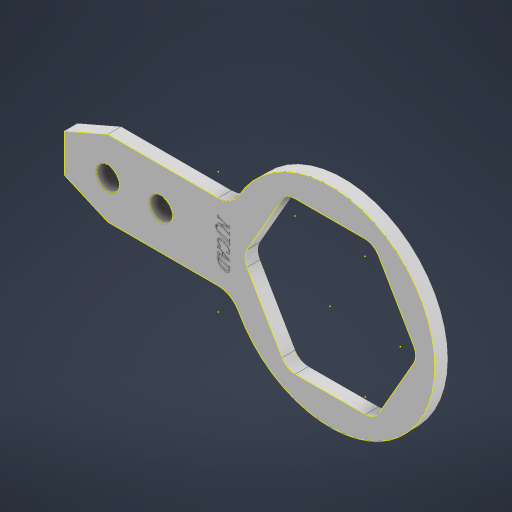
# Autodesk Inventor part: BICYCLE SPANNER
Saved by Autodesk Inventor 2023 (Build 270158000, 158)
## iProperties
Created: 2024-01-19
Part Number: BICYCLE SPANNER
Material: Generic
Document SubType Name: Modeling
Designer: User
Density: 1 g/cm^3
Appearance: Default
Author: User
Autodesk Inventor part; units mm, degrees
ref_plane "YZ Plane" through (0, 0, 0) normal (1, 0, 0) x (0, 1, 0)
ref_plane "XZ Plane" through (0, 0, 0) normal (0, 1, 0) x (-1, 0, 0)
ref_plane "XY Plane" through (0, 0, 0) normal (0, 0, 1) x (1, 0, 0)
sketch "Sketch1" plane through (0, 0, 0) normal (0, 0, 1) x (1, 0, 0)
  line L0 (25.3172, 36.0607) -> (43.8689, 4.105)
  line L1 (43.8881, -3.8949) -> (25.4895, -35.9391)
  line L2 (18.5709, -39.9557) -> (-18.3794, -40.0441)
  line L3 (-25.3172, -36.0607) -> (-43.8689, -4.105)
  line L4 (-43.8881, 3.8949) -> (-25.4895, 35.9391)
  line L5 (-18.5709, 39.9557) -> (18.3794, 40.0441)
  arc A0 (-48.3214, -26.2687) -> (-48.3214, 26.2687) centre (0, 0) ccw
  line L6 (-58.8643, 20) -> (-117, 20)
  line L7 (-58.8643, -20) -> (-117, -20)
  line L8 (-140, 10) -> (-140, -10)
  line L9 (-140, 0) -> (0, 0) construction
  line L10 (-117, 20) -> (-140, 10)
  line L11 (-140, -10) -> (-117, -20)
  arc A1 (-58.8643, 20) -> (-48.3214, 26.2687) centre (-58.8643, 32) ccw
  arc A2 (-48.3214, -26.2687) -> (-58.8643, -20) centre (-58.8643, -32) ccw
  arc A3 (-18.5709, 39.9557) -> (-25.4895, 35.9391) centre (-18.5518, 31.9557) ccw
  arc A4 (25.3172, 36.0607) -> (18.3794, 40.0441) centre (18.3985, 32.0441) ccw
  arc A5 (-43.8881, 3.8949) -> (-43.8689, -4.105) centre (-36.9503, -0.0885) ccw
  arc A6 (43.8881, -3.8949) -> (43.8689, 4.105) centre (36.9503, 0.0885) ccw
  arc A7 (18.5709, -39.9557) -> (25.4895, -35.9391) centre (18.5518, -31.9557) ccw
  arc A8 (-25.3172, -36.0607) -> (-18.3794, -40.0441) centre (-18.3985, -32.0441) ccw
  circle A9 centre (-117, 0) radius 6
  circle A10 centre (-89, 0) radius 6
  point P0 (22.9982, 40.0552)
  point P1 (46.1879, 0.1106)
  point P2 (23.1897, -39.9446)
  point P3 (-22.9982, -40.0552)
  point P4 (-46.1879, -0.1106)
  point P5 (-23.1897, 39.9446)
  point P6 (-0.0958, 39.9999)
  point P7 (0.0958, -39.9999)
  point P8 (-51.2348, -20)
  point P9 (-51.2348, 20)
  dimension "d1" = 79.9998
  dimension "d2" = 80
  dimension "d3" = 110
  dimension "d4" = 20
  dimension "d5" = 140
  dimension "d6" = 40
  dimension "d10" = 12
  dimension "d11" = 8
  dimension "d12" = 12
  dimension "d13" = 23
  dimension "d14" = 28
  constraints: 24 end point, 20 point on circle, 16 point on line, 16 tangent, 11 centre point, 7 equal radius, 3 horizontal, 3 midpoint, 2 coincident, 2 vertical alignment, 1 horizontal alignment, 1 vertical, 14 other
  measures "d1" vertical distance of point (-0.096, 40) point (0.096, -40)
  measures "d2" distance of point (46.188, 0.111) point (-22.998, -40.055)
  measures "d3" diameter of A0
  measures "d4" distance of L8.start L8.end
  measures "d5" distance of L9.start point (0, 0)
  measures "d6" distance between parallel lines of L7 L6
  measures "d10" radius of A1
  measures "d11" radius of A3
  measures "d12" diameter of A9
  measures "d13" horizontal distance of A9.centre L8.end
  measures "d14" distance of A10.centre A9.centre
extrude "Extrusion1" add sketch "Sketch1" along normal blind 7
sketch "Sketch2" plane through (0, 0, 7) normal (0, 0, 1) x (1, 0, 0)
  arc A0 (-48.3214, -26.2687) -> (-48.3214, 26.2687) centre (0, 0) ccw projected
  arc A1 (-58.8643, 20) -> (-48.3214, 26.2687) centre (-58.8643, 32) ccw projected
  line L0 (-58.8643, 20) -> (-117, 20) projected
  line L1 (-117, 20) -> (-140, 10) projected
  line L2 (-140, 10) -> (-140, -10) projected
  line L3 (-140, -10) -> (-117, -20) projected
  line L4 (-117, -20) -> (-58.8643, -20) projected
  arc A2 (-48.3214, -26.2687) -> (-58.8643, -20) centre (-58.8643, -32) ccw projected
  line L5 (-18.5709, 39.9557) -> (18.3794, 40.0441) projected
  arc A3 (25.3172, 36.0607) -> (18.3794, 40.0441) centre (18.3985, 32.0441) ccw projected
  line L6 (25.3172, 36.0607) -> (43.8689, 4.105) projected
  arc A4 (43.8881, -3.8949) -> (43.8689, 4.105) centre (36.9503, 0.0885) ccw projected
  line L7 (43.8881, -3.8949) -> (25.4895, -35.9391) projected
  arc A5 (18.5709, -39.9557) -> (25.4895, -35.9391) centre (18.5518, -31.9557) ccw projected
  line L8 (18.5709, -39.9557) -> (-18.3794, -40.0441) projected
  arc A6 (-25.3172, -36.0607) -> (-18.3794, -40.0441) centre (-18.3985, -32.0441) ccw projected
  line L9 (-25.3172, -36.0607) -> (-43.8689, -4.105) projected
  arc A7 (-43.8881, 3.8949) -> (-43.8689, -4.105) centre (-36.9503, -0.0885) ccw projected
  line L10 (-43.8881, 3.8949) -> (-25.4895, 35.9391) projected
  arc A8 (-18.5709, 39.9557) -> (-25.4895, 35.9391) centre (-18.5518, 31.9557) ccw projected
  circle A9 centre (-89, 0) radius 6 projected
  circle A10 centre (-117, 0) radius 6 projected
sketch "Sketch4" plane through (0, 0, 7) normal (0, 0, 1) x (1, 0, 0)
  line L0 (-52.8304, 12.3394) -> (-52.8304, -11.579) construction
  line L1 (-52.8304, -11.579) -> (-60.2146, -11.579) construction
  line L2 (-60.2146, -11.579) -> (-60.2146, 12.3394) construction
  line L3 (-60.2146, 12.3394) -> (-52.8304, 12.3394) construction
  line L4 (-57.6462, 8.2014) -> (-57.6462, 8.13)
  line L5 (-57.6462, 8.13) -> (-53.4725, 6.712)
  spline S0 degree 2 poles (-53.4725, 6.712) (-53.3298, 6.663) (-53.1871, 6.7611) (-53.1871, 6.9395) knots 0 0 0 1 2 2 2
  line L6 (-53.1871, 6.9395) -> (-53.1871, 7.2248)
  line L7 (-53.1871, 7.2248) -> (-52.9731, 7.149)
  line L8 (-52.9731, 7.149) -> (-52.9731, 5.7221)
  line L9 (-52.9731, 5.7221) -> (-53.1871, 5.7979)
  line L10 (-53.1871, 5.7979) -> (-53.1871, 6.0833)
  spline S1 degree 2 poles (-53.1871, 6.0833) (-53.1871, 6.226) (-53.3298, 6.449) (-53.4725, 6.498) knots 0 0 0 1 2 2 2
  line L11 (-53.4725, 6.498) -> (-59.0731, 8.402)
  line L12 (-59.0731, 8.402) -> (-59.0731, 8.6161)
  line L13 (-59.0731, 8.6161) -> (-53.7579, 9.5213)
  line L14 (-53.7579, 9.5213) -> (-53.7579, 9.5926)
  line L15 (-53.7579, 9.5926) -> (-58.5737, 11.2291)
  spline S2 degree 2 poles (-58.5737, 11.2291) (-58.7163, 11.2781) (-58.859, 11.1488) (-58.859, 11.0061) knots 0 0 0 1 2 2 2
  line L16 (-58.859, 11.0061) -> (-58.859, 10.7207)
  line L17 (-58.859, 10.7207) -> (-59.0731, 10.7921)
  line L18 (-59.0731, 10.7921) -> (-59.0731, 12.219)
  line L19 (-59.0731, 12.219) -> (-58.859, 12.1476)
  line L20 (-58.859, 12.1476) -> (-58.859, 11.8623)
  spline S3 degree 2 poles (-58.859, 11.8623) (-58.859, 11.6839) (-58.7163, 11.4922) (-58.5737, 11.4431) knots 0 0 0 1 2 2 2
  line L21 (-58.5737, 11.4431) -> (-53.4725, 9.7085)
  spline S4 degree 2 poles (-53.4725, 9.7085) (-53.3298, 9.6595) (-53.1871, 9.7576) (-53.1871, 9.9359) knots 0 0 0 1 2 2 2
  line L22 (-53.1871, 9.9359) -> (-53.1871, 10.15)
  line L23 (-53.1871, 10.15) -> (-52.9731, 10.0742)
  line L24 (-52.9731, 10.0742) -> (-52.9731, 9.0397)
  line L25 (-52.9731, 9.0397) -> (-57.6462, 8.2014)
  spline S5 degree 2 poles (-53.4725, 3.2161) (-53.3298, 3.1671) (-53.1871, 3.2652) (-53.1871, 3.4436) knots 0 0 0 1 2 2 2
  line L26 (-53.1871, 3.4436) -> (-53.1871, 4.2997)
  line L27 (-53.1871, 4.2997) -> (-52.9731, 4.2239)
  line L28 (-52.9731, 4.2239) -> (-52.9731, 1.2987)
  line L29 (-52.9731, 1.2987) -> (-53.1871, 1.3745)
  line L30 (-53.1871, 1.3745) -> (-53.1871, 2.2307)
  spline S6 degree 2 poles (-53.1871, 2.2307) (-53.1871, 2.3734) (-53.3298, 2.5963) (-53.4725, 2.6454) knots 0 0 0 1 2 2 2
  line L31 (-53.4725, 2.6454) -> (-58.538, 4.3666)
  spline S7 degree 2 poles (-58.538, 4.3666) (-59.3228, 4.6341) (-60.2146, 5.9362) (-60.2146, 6.6853) knots 0 0 0 1 2 2 2
  spline S8 degree 2 poles (-60.2146, 6.6853) (-60.2146, 7.2204) (-59.7865, 7.644) (-59.5011, 7.5503) knots 0 0 0 1 2 2 2
  spline S9 degree 2 poles (-59.5011, 7.5503) (-59.2871, 7.4745) (-59.0731, 7.1535) (-59.0731, 7.0108) knots 0 0 0 1 2 2 2
  spline S10 degree 2 poles (-59.0731, 7.0108) (-59.0731, 6.8324) (-59.3228, 6.7031) (-59.5011, 6.7656) knots 0 0 0 1 2 2 2
  spline S11 degree 2 poles (-59.5011, 6.7656) (-59.5725, 6.7878) (-59.6795, 6.8592) (-59.7509, 6.9573) knots 0 0 0 1 2 2 2
  spline S12 degree 2 poles (-59.7509, 6.9573) (-59.8579, 6.9216) (-59.9649, 6.6719) (-59.9649, 6.4579) knots 0 0 0 1 2 2 2
  spline S13 degree 2 poles (-59.9649, 6.4579) (-59.9649, 5.9941) (-59.3585, 5.2183) (-58.538, 4.9373) knots 0 0 0 1 2 2 2
  line L32 (-58.538, 4.9373) -> (-53.4725, 3.2161)
  spline S14 degree 2 poles (-59.1444, 0.7235) (-59.1444, 1.7224) (-57.6462, 2.3868) (-56.0409, 1.8427) knots 0 0 0 1 2 2 2
  spline S15 degree 2 poles (-56.0409, 1.8427) (-54.6854, 1.3835) (-52.9017, -0.4715) (-52.9017, -1.5417) knots 0 0 0 1 2 2 2
  spline S16 degree 2 poles (-52.9017, -1.5417) (-52.9017, -1.7914) (-52.9731, -2.0188) knots 0 0 0 1 1 1
  spline S17 degree 2 poles (-52.9731, -2.0188) (-53.0801, -2.2328) (-53.0801, -2.4112) knots 0 0 0 1 1 1
  spline S18 degree 2 poles (-53.0801, -2.4112) (-53.0801, -2.5539) (-53.0087, -2.7545) (-52.9017, -2.8616) knots 0 0 0 1 2 2 2
  line L33 (-52.9017, -2.8616) -> (-54.4713, -2.652)
  line L34 (-54.4713, -2.652) -> (-54.5427, -2.4112)
  spline S19 degree 2 poles (-54.5427, -2.4112) (-53.8649, -2.429) (-53.1514, -1.9564) (-53.1514, -1.3856) knots 0 0 0 1 2 2 2
  spline S20 degree 2 poles (-53.1514, -1.3856) (-53.1514, -0.6365) (-54.7924, 0.7414) (-56.0052, 1.1516) knots 0 0 0 1 2 2 2
  spline S21 degree 2 poles (-56.0052, 1.1516) (-57.3251, 1.602) (-58.8234, 1.3968) (-58.8234, 0.5764) knots 0 0 0 1 2 2 2
  spline S22 degree 2 poles (-58.8234, 0.5764) (-58.8234, 0.0056) (-58.0029, -1.0913) (-57.3251, -1.4659) knots 0 0 0 1 2 2 2
  line L35 (-57.3251, -1.4659) -> (-57.4321, -1.6442)
  spline S23 degree 2 poles (-57.4321, -1.6442) (-58.1813, -1.2117) (-59.1444, 0.0814) (-59.1444, 0.7235) knots 0 0 0 1 2 2 2
  line L36 (-56.79, -5.0733) -> (-56.79, -3.468)
  line L37 (-56.79, -3.468) -> (-58.1456, -2.6877)
  spline S24 degree 2 poles (-58.1456, -2.6877) (-58.3239, -2.5896) (-58.431, -2.5539) knots 0 0 0 1 1 1
  spline S25 degree 2 poles (-58.431, -2.5539) (-58.5737, -2.5048) (-58.859, -2.5138) (-58.859, -2.7635) knots 0 0 0 1 2 2 2
  line L38 (-58.859, -2.7635) -> (-58.859, -2.8705)
  line L39 (-58.859, -2.8705) -> (-59.0731, -2.7991)
  line L40 (-59.0731, -2.7991) -> (-59.0731, -1.4793)
  line L41 (-59.0731, -1.4793) -> (-58.859, -1.5506)
  line L42 (-58.859, -1.5506) -> (-58.859, -1.6576)
  spline S26 degree 2 poles (-58.859, -1.6576) (-58.859, -1.8003) (-58.6807, -2.0768) (-58.4666, -2.1838) knots 0 0 0 1 2 2 2
  line L43 (-58.4666, -2.1838) -> (-53.0087, -5.43)
  line L44 (-53.0087, -5.43) -> (-52.8304, -6.0275)
  line L45 (-52.8304, -6.0275) -> (-58.4666, -5.4657)
  spline S27 degree 2 poles (-58.4666, -5.4657) (-58.6807, -5.4657) (-58.859, -5.6173) (-58.859, -5.76) knots 0 0 0 1 2 2 2
  line L46 (-58.859, -5.76) -> (-58.859, -5.867)
  line L47 (-58.859, -5.867) -> (-59.0731, -5.7956)
  line L48 (-59.0731, -5.7956) -> (-59.0731, -4.2617)
  line L49 (-59.0731, -4.2617) -> (-58.859, -4.3331)
  line L50 (-58.859, -4.3331) -> (-58.859, -4.4757)
  spline S28 degree 2 poles (-58.859, -4.4757) (-58.859, -4.6898) (-58.6807, -4.8236) (-58.6093, -4.8459) knots 0 0 0 1 2 2 2
  spline S29 degree 2 poles (-58.6093, -4.8459) (-58.4666, -4.8949) (-58.3596, -4.8949) knots 0 0 0 1 1 1
  line L51 (-58.3596, -4.8949) -> (-56.79, -5.0733)
  line L52 (-53.6152, -5.4032) -> (-53.6152, -5.3676)
  line L53 (-53.6152, -5.3676) -> (-56.576, -3.6107)
  line L54 (-56.576, -3.6107) -> (-56.576, -5.1089)
  line L55 (-56.576, -5.1089) -> (-53.6152, -5.4032)
  spline S30 degree 2 poles (-53.4725, -8.6271) (-53.3298, -8.6762) (-53.1871, -8.5781) (-53.1871, -8.3997) knots 0 0 0 1 2 2 2
  line L56 (-53.1871, -8.3997) -> (-53.1871, -8.1857)
  line L57 (-53.1871, -8.1857) -> (-52.9731, -8.2615)
  line L58 (-52.9731, -8.2615) -> (-52.9731, -9.8668)
  spline S31 degree 2 poles (-52.9731, -9.8668) (-52.9731, -10.9726) (-54.4, -11.8064) (-55.8982, -11.2981) knots 0 0 0 1 2 2 2
  spline S32 degree 2 poles (-55.8982, -11.2981) (-57.5392, -10.7407) (-59.0731, -8.9348) (-59.0731, -7.6863) knots 0 0 0 1 2 2 2
  line L59 (-59.0731, -7.6863) -> (-59.0731, -6.1524)
  line L60 (-59.0731, -6.1524) -> (-58.859, -6.2237)
  line L61 (-58.859, -6.2237) -> (-58.859, -6.4734)
  spline S33 degree 2 poles (-58.859, -6.4734) (-58.859, -6.6518) (-58.7163, -6.8435) (-58.5737, -6.8926) knots 0 0 0 1 2 2 2
  line L62 (-58.5737, -6.8926) -> (-53.4725, -8.6271)
  spline S34 degree 2 poles (-55.9696, -10.5936) (-54.4356, -11.1153) (-53.1871, -10.6114) (-53.1871, -9.791) knots 0 0 0 1 2 2 2
  spline S35 degree 2 poles (-53.1871, -9.791) (-53.1871, -9.5412) (-53.3298, -9.2469) (-53.4725, -9.1979) knots 0 0 0 1 2 2 2
  line L63 (-53.4725, -9.1979) -> (-58.5737, -7.4633)
  spline S36 degree 2 poles (-58.5737, -7.4633) (-58.7163, -7.4143) (-58.859, -7.5793) (-58.859, -7.7576) knots 0 0 0 1 2 2 2
  spline S37 degree 2 poles (-58.859, -7.7576) (-58.859, -8.5424) (-57.6818, -10.0139) (-55.9696, -10.5936) knots 0 0 0 1 2 2 2
  point P0 (0, 0)
  constraints: 2 other
emboss "Emboss2" sketch "Sketch4" operation cut depth 1 direction (0, 0, -1)
body "Solid1"
